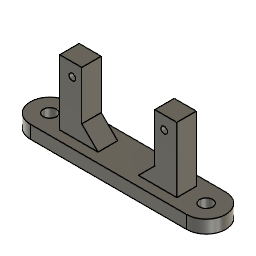
Servo Mount (Autodesk Fusion 360 design; units mm, degrees)
Autodesk Fusion 360 part; units mm, degrees
sketch "Sketch1" plane through (0, 0, 0) normal (0, 1, 0) x (1, 0, 0)
  line L0 (-30, 0) -> (30, 0)
  line L1 (30, 0) -> (30, -4)
  line L2 (30, -4) -> (-30, -4)
  line L3 (-30, -4) -> (-30, 0)
  line L4 (-18, -4) -> (-11.2, -4)
  line L5 (-11.2, -4) -> (-11.2, -24)
  line L6 (-11.2, -24) -> (-18, -24)
  line L7 (-18, -24) -> (-18, -4)
  circle A0 centre (-14.1, -20) radius 1
  line L8 (0, -20) -> (0, -2.5)
  line L9 (11.2, -24) -> (18, -24)
  line L10 (11.2, -4) -> (11.2, -24)
  line L11 (18, -24) -> (18, -4)
  circle A1 centre (14.1, -20) radius 1
  dimension "d1" = 4
  dimension "d2" = 60
  dimension "d3" = 6.8
  dimension "d4" = 30
  dimension "d5" = 18
  dimension "d6" = 20
  dimension "d7" = 2
  dimension "d8" = 2.9
  dimension "d9" = 4
  dimension "d10" = 4
  constraint horizontal L0
  constraint vertical L1
  constraint horizontal L2
  constraint vertical L3
  constraint horizontal L4
  constraint vertical L5
  constraint horizontal L6
  constraint vertical L7
  constraint coincident L2 L4.start
  constraint symmetric L4.start L8 L11.end
  constraint symmetric L4.end L8 L10.start
  constraint symmetric L5.end L8 L9.start
  constraint symmetric L6.end L8 L9.end
  constraint symmetric A0 L8 A1
  measures "d1" distance of L0.start L2.end
  measures "d2" distance of L0.start L0.end
  measures "d3" distance of L5.end L6.end
  measures "d4" distance of origin L3
  measures "d5" distance of origin L7
  measures "d6" distance of L4.start L6.end
  measures "d7" diameter of A0
  measures "d8" distance of L5 A0.centre
  measures "d9" distance of L6 A0.centre
  measures "d10" distance of origin L2
extrude "Extrude1" add sketch "Sketch1" along normal blind 12 contours L0 L1 L2 L3 L4
extrude "Extrude2" add sketch "Sketch1" along normal blind 9 and the other way blind -3 contours L2 L4 L5 L6 L7 | L2 L9 L10 L11
chamfer "Chamfer1" distance 5 angle 45 2 edges at (-11.2, 6, 4) (11.2, 6, 4)
sketch "Sketch2" plane through (0, 0, 0) normal (0, 0, 1) x (1, 0, 0)
  circle A0 centre (-24, 6) radius 2
  line L0 (0, 2.5) -> (0, 20)
  circle A1 centre (24, 6) radius 2
  dimension "d18" = 4
  dimension "d19" = 24
  dimension "d20" = 6
  constraint symmetric A0 L0 A1
  measures "d18" diameter of A0
  measures "d19" horizontal distance of origin A0.centre
  measures "d20" vertical distance of origin A0.centre
extrude "Extrude3" cut sketch "Sketch2" along normal blind 10
fillet "Fillet1" radius 6 4 edges at (-30, 0, 2) (30, 0, 2) (30, 12, 2) (-30, 12, 2)
equation "d4 = d2 / 2"
equation "d10 = d1"
